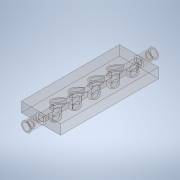
# Autodesk Inventor part: 1stGenValve
Saved by Autodesk Inventor 2020 (Build 240168000, 168)
## iProperties
Created: 2019-11-21
Part Number: 1stGenValve
Material: Glass, Cast, Gray
Document SubType Name: Modeling
Designer: chuff
Density: 2.18 g/cm^3
Appearance: Dark Gray
Author: chuff
Autodesk Inventor part; units mm, degrees
ref_plane "YZ Plane" through (0, 0, 0) normal (1, 0, 0) x (0, 1, 0)
ref_plane "XZ Plane" through (0, 0, 0) normal (0, 1, 0) x (-1, 0, 0)
ref_plane "XY Plane" through (0, 0, 0) normal (0, 0, 1) x (1, 0, 0)
sketch "Sketch1" plane through (0, 0, 0) normal (0, 1, 0) x (-1, 0, 0)
  line L0 (0, 0) -> (-20, 0)
  line L1 (-20, 0) -> (-20, -20)
  line L2 (-20, -20) -> (0, -20)
  line L3 (0, -20) -> (0, 0)
  dimension "d0" = 20
  dimension "d1" = 20
  constraints: 8 end point, 2 parallel, 1 horizontal, 1 perpendicular
  measures "d0" distance of L2.end L1.end
  measures "d1" distance of L1.end L0.end
extrude "Extrusion1" add sketch "Sketch1" along normal blind 1.5
sketch "Sketch3" plane through (0, 1.5, 0) normal (0, 1, 0) x (1, 0, 0)
  line L0 (0, 0) -> (20, 0) projected
  line L1 (10, 0) -> (10, 20)
  line L2 (20, 20) -> (0, 20) projected
  line L3 (10, 0) -> (10.5, 0)
  line L4 (10, 0) -> (9.5, 0)
  line L5 (9.5, 0) -> (9, 0)
  line L6 (10.5, 0) -> (11, 0)
  line L7 (9, 0) -> (9, 20)
  line L8 (11, 0) -> (11, 20)
  line L9 (10.5, 0) -> (10.5, 20)
  line L10 (9.5, 0) -> (9.5, 20)
  line L11 (10, 0) -> (10, 1)
  line L12 (10, 20) -> (10, 19)
  line L13 (10, 19) -> (10, 17)
  line L14 (10, 17) -> (10, 15)
  line L15 (10, 15) -> (10, 13)
  line L16 (10, 13) -> (10, 11)
  line L17 (10, 11) -> (10, 9)
  line L18 (10, 9) -> (10, 7)
  line L19 (10, 7) -> (10, 5)
  line L20 (10, 5) -> (10, 3)
  line L21 (10, 3) -> (10, 1)
  line L22 (10, 3) -> (10, 1)
  ellipse E0 centre (9, 4.13) end of major axis (8.8201, 3.4422) minor radius 0.2643
  ellipse E1 centre (9, 8) end of major axis (8.8201, 7.3122) minor radius 0.2643
  ellipse E2 centre (9, 12) end of major axis (8.8201, 11.3122) minor radius 0.2643
  ellipse E3 centre (9, 16) end of major axis (8.8201, 15.3122) minor radius 0.2643
  ellipse E4 centre (11, 14) end of major axis (11.1799, 13.3122) minor radius 0.2643
  ellipse E5 centre (11, 10) end of major axis (11.1799, 9.3122) minor radius 0.2643
  ellipse E6 centre (11, 6) end of major axis (11.1799, 5.3122) minor radius 0.2643
  ellipse E7 centre (11, 2) end of major axis (11.1799, 1.3122) minor radius 0.2643
  ellipse E8 centre (11, 18) end of major axis (11.1799, 17.3122) minor radius 0.2643
  line L23 (10.5, 1.0973) -> (11.1799, 0.7881) construction
  line L24 (11.1799, 0.7881) -> (11.8108, 1.1878) construction
  line L25 (11.8108, 1.1878) -> (12.1124, 1.8289) construction
  line L26 (12.1124, 1.8289) -> (11.4413, 2.9601) construction
  line L27 (11.4413, 2.9601) -> (10.5, 3.6087) construction
  spline S0 degree 4 poles (10.5, 1.0973) (11.1799, 0.7881) (11.8108, 1.1878) (12.1124, 1.8289) (11.4413, 2.9601) (10.5, 3.6087) knots 1 1 1 1 1 2 3 3 3 3 3
  line L28 (10.482, 5.171) -> (11.1619, 4.8618) construction
  line L29 (11.1619, 4.8618) -> (11.7928, 5.2615) construction
  line L30 (11.7928, 5.2615) -> (12.0945, 5.9025) construction
  line L31 (12.0945, 5.9025) -> (11.4233, 7.0337) construction
  line L32 (11.4233, 7.0337) -> (10.482, 7.6823) construction
  spline S1 degree 4 poles (10.482, 5.171) (11.1619, 4.8618) (11.7928, 5.2615) (12.0945, 5.9025) (11.4233, 7.0337) (10.482, 7.6823) knots 1 1 1 1 1 2 3 3 3 3 3
  line L33 (10.4828, 9.0005) -> (11.1627, 8.6913) construction
  line L34 (11.1627, 8.6913) -> (11.7936, 9.091) construction
  line L35 (11.7936, 9.091) -> (12.0952, 9.732) construction
  line L36 (12.0952, 9.732) -> (11.424, 10.8633) construction
  line L37 (11.424, 10.8633) -> (10.4828, 11.5118) construction
  spline S2 degree 4 poles (10.4828, 9.0005) (11.1627, 8.6913) (11.7936, 9.091) (12.0952, 9.732) (11.424, 10.8633) (10.4828, 11.5118) knots 1 1 1 1 1 2 3 3 3 3 3
  line L38 (10.491, 12.9429) -> (11.1709, 12.6337) construction
  line L39 (11.1709, 12.6337) -> (11.8018, 13.0334) construction
  line L40 (11.8018, 13.0334) -> (12.1034, 13.6744) construction
  line L41 (12.1034, 13.6744) -> (11.4322, 14.8056) construction
  line L42 (11.4322, 14.8056) -> (10.491, 15.4542) construction
  spline S3 degree 4 poles (10.491, 12.9429) (11.1709, 12.6337) (11.8018, 13.0334) (12.1034, 13.6744) (11.4322, 14.8056) (10.491, 15.4542) knots 1 1 1 1 1 2 3 3 3 3 3
  line L43 (10.497, 16.887) -> (11.1769, 16.5778) construction
  line L44 (11.1769, 16.5778) -> (11.8078, 16.9775) construction
  line L45 (11.8078, 16.9775) -> (12.1095, 17.6186) construction
  line L46 (12.1095, 17.6186) -> (11.4383, 18.7498) construction
  line L47 (11.4383, 18.7498) -> (10.497, 19.3984) construction
  spline S4 degree 4 poles (10.497, 16.887) (11.1769, 16.5778) (11.8078, 16.9775) (12.1095, 17.6186) (11.4383, 18.7498) (10.497, 19.3984) knots 1 1 1 1 1 2 3 3 3 3 3
  spline S5 degree 4 poles (9.5222, 3.1349) (8.8424, 2.8257) (8.2115, 3.2254) (7.9098, 3.8664) (8.581, 4.9976) (9.5222, 5.6462) knots 1 1 1 1 1 2 3 3 3 3 3
  line L48 (9.5222, 3.1349) -> (8.8424, 2.8257) construction
  line L49 (8.8424, 2.8257) -> (8.2115, 3.2254) construction
  line L50 (8.2115, 3.2254) -> (7.9098, 3.8664) construction
  line L51 (7.9098, 3.8664) -> (8.581, 4.9976) construction
  line L52 (8.581, 4.9976) -> (9.5222, 5.6462) construction
  spline S6 degree 4 poles (9.5114, 6.9421) (8.8315, 6.6329) (8.2006, 7.0326) (7.8989, 7.6736) (8.5701, 8.8048) (9.5114, 9.4534) knots 1 1 1 1 1 2 3 3 3 3 3
  line L53 (9.5114, 6.9421) -> (8.8315, 6.6329) construction
  line L54 (8.8315, 6.6329) -> (8.2006, 7.0326) construction
  line L55 (8.2006, 7.0326) -> (7.8989, 7.6736) construction
  line L56 (7.8989, 7.6736) -> (8.5701, 8.8048) construction
  line L57 (8.5701, 8.8048) -> (9.5114, 9.4534) construction
  spline S7 degree 4 poles (9.5213, 10.9708) (8.8414, 10.6616) (8.2105, 11.0613) (7.9089, 11.7023) (8.5801, 12.8335) (9.5213, 13.4821) knots 1 1 1 1 1 2 3 3 3 3 3
  line L58 (9.5213, 10.9708) -> (8.8414, 10.6616) construction
  line L59 (8.8414, 10.6616) -> (8.2105, 11.0613) construction
  line L60 (8.2105, 11.0613) -> (7.9089, 11.7023) construction
  line L61 (7.9089, 11.7023) -> (8.5801, 12.8335) construction
  line L62 (8.5801, 12.8335) -> (9.5213, 13.4821) construction
  spline S8 degree 4 poles (9.5157, 14.8194) (8.8359, 14.5102) (8.205, 14.9099) (7.9033, 15.551) (8.5745, 16.6822) (9.5157, 17.3308) knots 1 1 1 1 1 2 3 3 3 3 3
  line L63 (9.5157, 14.8194) -> (8.8359, 14.5102) construction
  line L64 (8.8359, 14.5102) -> (8.205, 14.9099) construction
  line L65 (8.205, 14.9099) -> (7.9033, 15.551) construction
  line L66 (7.9033, 15.551) -> (8.5745, 16.6822) construction
  line L67 (8.5745, 16.6822) -> (9.5157, 17.3308) construction
  point P0 (10.5, 7.6699)
  point P1 (10.5, 8.9928)
  point P2 (10.5, 11.4999)
  point P3 (10.5, 12.9388)
  point P4 (10.5, 15.448)
  point P5 (10.5, 16.8857)
  point P6 (10.5, 19.3963)
  point P7 (9.5, 17.3199)
  point P8 (9.5, 14.8124)
  point P9 (9.5, 13.4673)
  point P10 (9.5, 10.9612)
  point P11 (9.5, 9.4455)
  point P12 (9.5, 6.9369)
  point P13 (9.5, 5.6308)
  point P14 (9.5, 3.1249)
  point P15 (10.5, 5.1629)
  constraints: 40 end point, 18 point on line, 5 centre point, 3 midpoint, 2 vertical, 1 perpendicular, 48 other
extrude "Extrusion2" cut sketch "Sketch3" against normal blind 1 contours L10 L2 L1 L0 | S5 L7 E0 | L7 E0 S5 L10 | L1 L2 L9 L0 | S6 L7 E1 | L7 E1 S6 L10 | L9 S0 L8 E7 | L8 E7 S0 | S7 L7 E2 | L7 E2 S7 L10 | L9 S1 L8 E6 | L8 E6 S1 | S8 L7 E3 | L7 E3 S8 L10 | L9 S2 L8 E5 | L8 E5 S2 | L9 S3 L8 E4 | L8 E4 S3 | L9 S4 L8 E8 | L8 E8 S4
sketch "Sketch5" plane through (0, 1.5, 0) normal (0, 1, 0) x (1, 0, 0)
  ellipse E0 centre (9.1164, 8.1584) end of major axis (8.6253, 7.1754) minor radius 0.4202
  ellipse E1 centre (9.1164, 4.3477) end of major axis (8.6253, 3.3647) minor radius 0.4202
  ellipse E2 centre (9.1164, 12.1855) end of major axis (8.6253, 11.2025) minor radius 0.4202
  ellipse E3 centre (9.1164, 16.0098) end of major axis (8.6253, 15.0268) minor radius 0.4202
  ellipse E4 centre (10.8106, 18.0711) end of major axis (11.3018, 17.0881) minor radius 0.4202
  ellipse E5 centre (10.8106, 14.1694) end of major axis (11.3018, 13.1864) minor radius 0.4202
  ellipse E6 centre (13.9856, 21.3528) end of major axis (14.4768, 20.3698) minor radius 0.4202
  ellipse E7 centre (15.5731, 22.9403) end of major axis (16.0643, 21.9573) minor radius 0.4202
  ellipse E8 centre (10.8106, 10.1967) end of major axis (11.3018, 9.2138) minor radius 0.4202
  ellipse E9 centre (10.8106, 6.3159) end of major axis (11.3018, 5.3329) minor radius 0.4202
  ellipse E10 centre (10.8106, 2.256) end of major axis (11.3018, 1.273) minor radius 0.4202
  point P0 (0, 0)
  constraints: 7 centre point, 8 other
extrude "Extrusion3" add sketch "Sketch5" against normal blind 1 contours E0 | E1 | E2 | E3 | E4 | E5 | E8 | E9 | E10
sketch "Sketch6" plane through (0, 1.5, 0) normal (0, 1, 0) x (1, 0, 0)
  line L0 (0, 0) -> (9.5, 0) projected
  line L1 (20, 20) -> (10.5, 20) projected
  line L2 (0, 0) -> (20, 0)
  line L3 (20, 0) -> (20, 20)
  line L4 (20, 20) -> (0, 20)
  line L5 (0, 20) -> (0, 0)
  constraints: 8 end point, 2 parallel, 1 horizontal, 1 perpendicular
extrude "Extrusion4" add sketch "Sketch6" along normal blind 0.5
sketch "Sketch8" plane through (0, 2, 0) normal (0, 1, 0) x (1, 0, 0)
  line L0 (20, 20) -> (0, 20) projected
  line L1 (20, 0) -> (14, 0)
  line L2 (14, 0) -> (14, 20)
  line L3 (14, 20) -> (20, 20)
  line L4 (20, 20) -> (20, 0)
  line L5 (0, 20) -> (0, 0) projected
  line L6 (0, 0) -> (6, 0)
  line L7 (6, 0) -> (6, 20)
  line L8 (6, 20) -> (0, 20)
  line L9 (0, 20) -> (0, 0)
  dimension "d32" = 6
  dimension "d33" = 6
  constraints: 16 end point, 4 parallel, 2 horizontal, 2 perpendicular, 2 point on line
  measures "d32" distance of L2.end L3.end
  measures "d33" distance of L8.end L7.end
extrude "Extrusion6" cut sketch "Sketch8" against normal blind 3
sketch "Sketch10" plane through (14, 0, -20) normal (0, 0, -1) x (-1, 0, 0)
  line L0 (0, 0) -> (8, 0) projected
  line L1 (4, 0) -> (4, 1)
  circle A0 centre (4, 1) radius 0.5
  line L2 (3.5, 1.5) -> (4.5, 1.5) projected
  circle A1 centre (4, 1) radius 1
  point P0 (14, 0)
  dimension "d36" = 1
  dimension "d37" = 2
  constraints: 2 centre point, 2 coincident, 2 end point, 1 midpoint, 1 tangent, 1 vertical
  measures "d36" distance of L1.start L1.end
  measures "d37" diameter of A1
extrude "Extrusion7" add sketch "Sketch10" along normal blind 3
sketch "Sketch13" plane through (10, 1, -23) normal (0, 0, -1) x (-1, 0, 0)
  circle A0 centre (0, 0) radius 0.7379
  point P0 (10, -1)
  constraints: 1 centre point
extrude "Extrusion8" cut sketch "Sketch13" against normal blind 1
sketch "Sketch15" plane through (6, 0, 0) normal (0, 0, 1) x (1, 0, 0)
  line L0 (3.5, 1.5) -> (4.5, 1.5) projected
  line L1 (4, 1.5) -> (4, 1)
  circle A0 centre (4, 1) radius 0.5
  circle A1 centre (4, 1) radius 1
  point P0 (-6, 0)
  dimension "d42" = 0.5
  dimension "d43" = 1
  dimension "d44" = 2
  constraints: 2 centre point, 2 coincident, 2 end point, 1 midpoint, 1 vertical
  measures "d42" distance of L1.start L1.end
  measures "d43" diameter of A0
  measures "d44" diameter of A1
extrude "Extrusion9" add sketch "Sketch15" along normal blind 3
sketch "Sketch17" plane through (10, 1, 3) normal (0, 0, 1) x (1, 0, 0)
  arc A0 (0, -0.5) -> (0.5, 0) centre (0, 0) ccw projected
  circle A1 centre (0, 0) radius 0.75
  point P0 (-10, -1)
  dimension "d47" = 1.5
  constraints: 1 centre point, 1 coincident
  measures "d47" diameter of A1
extrude "Extrusion10" cut sketch "Sketch17" against normal blind 1
body "Solid1"
